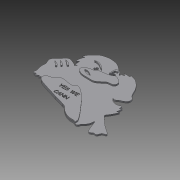
# Autodesk Inventor part: logo
Saved by Autodesk Inventor 2014 SP1 (Build 180222100, 222)
## iProperties
Created: 2015-10-19
Part Number: logo
Material: Generic
Document SubType Name: Modeling
Designer: Clayton
Density: 1 g/cm^3
Appearance: Default
Author: Clayton
Autodesk Inventor part; units mm, degrees
(part 1 of 2)
ref_plane "YZ Plane" through (0, 0, 0) normal (1, 0, 0) x (0, 1, 0)
ref_plane "XZ Plane" through (0, 0, 0) normal (0, 1, 0) x (-1, 0, 0)
ref_plane "XY Plane" through (0, 0, 0) normal (0, 0, 1) x (1, 0, 0)
sketch "Sketch1" plane through (0, 0, 0) normal (0, 1, 0) x (-1, 0, 0)
  line L0 (205.3182, -105.8082) -> (14.8182, -105.8082) construction
  line L1 (14.8182, -105.8082) -> (14.8182, 35.7439) construction
  line L2 (14.8182, 35.7439) -> (205.3182, 35.7439) construction
  line L3 (205.3182, 35.7439) -> (205.3182, -105.8082) construction
  line L4 (119.6658, -99.1182) -> (125.0217, -103.8066) construction
  line L5 (125.0217, -103.8066) -> (133.3036, -105.4948) construction
  line L6 (133.3036, -105.4948) -> (139.5998, -105.8082) construction
  line L7 (139.5998, -105.8082) -> (142.3045, -105.8082) construction
  line L8 (142.3045, -105.8082) -> (145.8288, -105.2062) construction
  line L9 (145.8288, -105.2062) -> (149.5668, -104.1037) construction
  line L10 (149.5668, -104.1037) -> (153.0365, -103.4823) construction
  line L11 (153.0365, -103.4823) -> (156.2624, -101.346) construction
  line L12 (156.2624, -101.346) -> (158.2697, -99.538) construction
  line L13 (158.2697, -99.538) -> (160.1706, -97.7361) construction
  line L14 (160.1706, -97.7361) -> (161.546, -96.1826) construction
  line L15 (161.546, -96.1826) -> (163.2097, -94.5009) construction
  line L16 (163.2097, -94.5009) -> (165.0974, -92.3655) construction
  line L17 (165.0974, -92.3655) -> (166.0638, -91.0856) construction
  line L18 (166.0638, -91.0856) -> (167.5222, -88.5574) construction
  line L19 (167.5222, -88.5574) -> (168.3582, -86.9182) construction
  line L20 (168.3582, -86.9182) -> (169.2598, -85.5249) construction
  line L21 (169.2598, -85.5249) -> (169.4073, -84.6889) construction
  line L22 (169.4073, -84.6889) -> (168.809, -84.5926) construction
  line L23 (168.809, -84.5926) -> (168.0493, -85.2715) construction
  line L24 (168.0493, -85.2715) -> (167.2824, -85.5249) construction
  line L25 (167.2824, -85.5249) -> (166.0912, -85.7774) construction
  line L26 (166.0912, -85.7774) -> (165.3732, -85.7774) construction
  spline S0 degree 4 poles (119.6658, -99.1182) (125.0217, -103.8066) (133.3036, -105.4948) (139.5998, -105.8082) (142.3045, -105.8082) (145.8288, -105.2062) (149.5668, -104.1037) (153.0365, -103.4823) (156.2624, -101.346) (158.2697, -99.538) (160.1706, -97.7361) (161.546, -96.1826) (163.2097, -94.5009) (165.0974, -92.3655) (166.0638, -91.0856) (167.5222, -88.5574) (168.3582, -86.9182) (169.2598, -85.5249) (169.4073, -84.6889) (168.809, -84.5926) (168.0493, -85.2715) (167.2824, -85.5249) (166.0912, -85.7774) (165.3732, -85.7774) knots 1 1 1 1 1 2 3 4 5 6 7 8 9 10 11 12 13 14 15 16 17 18 19 20 21 21 21 21 21
  line L27 (72.0061, 24.2829) -> (70.6525, 24.5535) construction
  line L28 (70.6525, 24.5535) -> (69.4998, 24.2136) construction
  line L29 (69.4998, 24.2136) -> (68.435, 23.4099) construction
  line L30 (68.435, 23.4099) -> (67.5909, 22.3816) construction
  line L31 (67.5909, 22.3816) -> (67.4318, 21.4798) construction
  line L32 (67.4318, 21.4798) -> (67.1775, 20.7659) construction
  line L33 (67.1775, 20.7659) -> (67.1345, 19.9018) construction
  line L34 (67.1345, 19.9018) -> (66.446, 19.2058) construction
  line L35 (66.446, 19.2058) -> (65.2763, 18.0971) construction
  line L36 (65.2763, 18.0971) -> (64.2775, 17.083) construction
  line L37 (64.2775, 17.083) -> (63.0251, 15.817) construction
  line L38 (63.0251, 15.817) -> (62.3988, 14.8491) construction
  line L39 (62.3988, 14.8491) -> (61.8964, 13.8641) construction
  line L40 (61.8964, 13.8641) -> (61.0497, 12.5555) construction
  line L41 (61.0497, 12.5555) -> (60.8463, 11.5383) construction
  line L42 (60.8463, 11.5383) -> (60.3804, 10.6247) construction
  line L43 (60.3804, 10.6247) -> (59.9183, 9.7186) construction
  line L44 (59.9183, 9.7186) -> (59.6793, 8.5233) construction
  line L45 (59.6793, 8.5233) -> (59.6041, 7.0137) construction
  line L46 (59.6041, 7.0137) -> (59.6041, 5.8018) construction
  line L47 (59.6041, 5.8018) -> (59.4165, 4.7385) construction
  line L48 (59.4165, 4.7385) -> (59.1255, 3.9217) construction
  line L49 (59.1255, 3.9217) -> (58.8425, 3.3668) construction
  line L50 (58.8425, 3.3668) -> (58.0971, 3.9787) construction
  line L51 (58.0971, 3.9787) -> (57.5959, 5.0609) construction
  line L52 (57.5959, 5.0609) -> (56.7878, 6.8058) construction
  line L53 (56.7878, 6.8058) -> (56.5067, 8.3755) construction
  line L54 (56.5067, 8.3755) -> (55.8124, 9.8748) construction
  spline S1 degree 4 poles (72.0061, 24.2829) (70.6525, 24.5535) (69.4998, 24.2136) (68.435, 23.4099) (67.5909, 22.3816) (67.4318, 21.4798) (67.1775, 20.7659) (67.1345, 19.9018) (66.446, 19.2058) (65.2763, 18.0971) (64.2775, 17.083) (63.0251, 15.817) (62.3988, 14.8491) (61.8964, 13.8641) (61.0497, 12.5555) (60.8463, 11.5383) (60.3804, 10.6247) (59.9183, 9.7186) (59.6793, 8.5233) (59.6041, 7.0137) (59.6041, 5.8018) (59.4165, 4.7385) (59.1255, 3.9217) (58.8425, 3.3668) (58.0971, 3.9787) (57.5959, 5.0609) (56.7878, 6.8058) (56.5067, 8.3755) (55.8124, 9.8748) knots 1 1 1 1 1 2 3 4 5 6 7 8 9 10 11 12 13 14 15 16 17 18 19 20 21 22 23 24 25 26 26 26 26 26
  line L55 (55.8124, 9.8748) -> (54.8371, 11.9808) construction
  line L56 (54.8371, 11.9808) -> (53.6125, 15.232) construction
  line L57 (53.6125, 15.232) -> (51.641, 19.9262) construction
  line L58 (51.641, 19.9262) -> (50.2656, 22.8961) construction
  line L59 (50.2656, 22.8961) -> (49.1599, 23.99) construction
  line L60 (49.1599, 23.99) -> (47.6368, 24.7667) construction
  line L61 (47.6368, 24.7667) -> (46.3346, 24.5335) construction
  line L62 (46.3346, 24.5335) -> (45.2431, 24.028) construction
  line L63 (45.2431, 24.028) -> (43.9979, 22.5111) construction
  line L64 (43.9979, 22.5111) -> (42.8586, 21.6512) construction
  line L65 (42.8586, 21.6512) -> (41.6778, 21.71) construction
  line L66 (41.6778, 21.71) -> (40.6321, 21.8548) construction
  line L67 (40.6321, 21.8548) -> (39.3449, 22.0819) construction
  line L68 (39.3449, 22.0819) -> (37.9514, 22.1513) construction
  line L69 (37.9514, 22.1513) -> (37.0993, 21.7566) construction
  line L70 (37.0993, 21.7566) -> (36.1467, 20.5961) construction
  line L71 (36.1467, 20.5961) -> (35.8442, 18.8823) construction
  line L72 (35.8442, 18.8823) -> (35.6072, 17.5392) construction
  line L73 (35.6072, 17.5392) -> (34.5467, 15.9002) construction
  line L74 (34.5467, 15.9002) -> (33.8767, 15.084) construction
  line L75 (33.8767, 15.084) -> (32.4017, 14.4009) construction
  line L76 (32.4017, 14.4009) -> (31.3382, 13.9084) construction
  line L77 (31.3382, 13.9084) -> (30.0361, 13.6752) construction
  line L78 (30.0361, 13.6752) -> (29.6443, 13.4938) construction
  line L79 (29.6443, 13.4938) -> (28.91, 12.5992) construction
  line L80 (28.91, 12.5992) -> (28.4728, 11.7419) construction
  line L81 (28.4728, 11.7419) -> (28.751, 11.1411) construction
  line L82 (28.751, 11.1411) -> (29.3294, 10.569) construction
  line L83 (29.3294, 10.569) -> (30.2816, 9.7873) construction
  line L84 (30.2816, 9.7873) -> (31.1945, 9.1966) construction
  spline S2 degree 4 poles (55.8124, 9.8748) (54.8371, 11.9808) (53.6125, 15.232) (51.641, 19.9262) (50.2656, 22.8961) (49.1599, 23.99) (47.6368, 24.7667) (46.3346, 24.5335) (45.2431, 24.028) (43.9979, 22.5111) (42.8586, 21.6512) (41.6778, 21.71) (40.6321, 21.8548) (39.3449, 22.0819) (37.9514, 22.1513) (37.0993, 21.7566) (36.1467, 20.5961) (35.8442, 18.8823) (35.6072, 17.5392) (34.5467, 15.9002) (33.8767, 15.084) (32.4017, 14.4009) (31.3382, 13.9084) (30.0361, 13.6752) (29.6443, 13.4938) (28.91, 12.5992) (28.4728, 11.7419) (28.751, 11.1411) (29.3294, 10.569) (30.2816, 9.7873) (31.1945, 9.1966) knots 1 1 1 1 1 2 3 4 5 6 7 8 9 10 11 12 13 14 15 16 17 18 19 20 21 22 23 24 25 26 27 28 28 28 28 28
  line L85 (31.1945, 9.1966) -> (41.8078, 2.3292) construction
  line L86 (41.8078, 2.3292) -> (46.7072, -2.0019) construction
  spline S3 degree 2 poles (31.1945, 9.1966) (41.8078, 2.3292) (46.7072, -2.0019) knots 1 1 1 2 2 2
  line L87 (46.7072, -2.0019) -> (51.207, -5.9799) construction
  line L88 (51.207, -5.9799) -> (53.5134, -8.2615) construction
  line L89 (53.5134, -8.2615) -> (55.9715, -10.8548) construction
  line L90 (55.9715, -10.8548) -> (58.4698, -13.0633) construction
  line L91 (58.4698, -13.0633) -> (60.1673, -14.7426) construction
  line L92 (60.1673, -14.7426) -> (59.1255, -16.3527) construction
  line L93 (59.1255, -16.3527) -> (57.769, -17.8873) construction
  line L94 (57.769, -17.8873) -> (55.4952, -21.8288) construction
  line L95 (55.4952, -21.8288) -> (53.9817, -24.1678) construction
  line L96 (53.9817, -24.1678) -> (52.5072, -27.5205) construction
  line L97 (52.5072, -27.5205) -> (51.6772, -29.4078) construction
  line L98 (51.6772, -29.4078) -> (50.8092, -31.8445) construction
  line L99 (50.8092, -31.8445) -> (50.6239, -32.8941) construction
  line L100 (50.6239, -32.8941) -> (51.5624, -32.4595) construction
  line L101 (51.5624, -32.4595) -> (52.7167, -31.6951) construction
  line L102 (52.7167, -31.6951) -> (54.3148, -30.839) construction
  line L103 (54.3148, -30.839) -> (54.927, -30.839) construction
  line L104 (54.927, -30.839) -> (54.5168, -32.8908) construction
  line L105 (54.5168, -32.8908) -> (53.7795, -34.9605) construction
  line L106 (53.7795, -34.9605) -> (53.9987, -36.9223) construction
  line L107 (53.9987, -36.9223) -> (53.9987, -39.207) construction
  line L108 (53.9987, -39.207) -> (53.9987, -39.8781) construction
  line L109 (53.9987, -39.8781) -> (54.1947, -40.9729) construction
  line L110 (54.1947, -40.9729) -> (54.9689, -39.7764) construction
  line L111 (54.9689, -39.7764) -> (56.2034, -38.1415) construction
  line L112 (56.2034, -38.1415) -> (57.0827, -37.4778) construction
  line L113 (57.0827, -37.4778) -> (56.9666, -39.8108) construction
  line L114 (56.9666, -39.8108) -> (57.2605, -42.4419) construction
  line L115 (57.2605, -42.4419) -> (57.2605, -44.4702) construction
  line L116 (57.2605, -44.4702) -> (60.64, -42.8559) construction
  line L117 (60.64, -42.8559) -> (62.1808, -42.1423) construction
  spline S4 degree 4 poles (46.7072, -2.0019) (51.207, -5.9799) (53.5134, -8.2615) (55.9715, -10.8548) (58.4698, -13.0633) (60.1673, -14.7426) (59.1255, -16.3527) (57.769, -17.8873) (55.4952, -21.8288) (53.9817, -24.1678) (52.5072, -27.5205) (51.6772, -29.4078) (50.8092, -31.8445) (50.6239, -32.8941) (51.5624, -32.4595) (52.7167, -31.6951) (54.3148, -30.839) (54.927, -30.839) (54.5168, -32.8908) (53.7795, -34.9605) (53.9987, -36.9223) (53.9987, -39.207) (53.9987, -39.8781) (54.1947, -40.9729) (54.9689, -39.7764) (56.2034, -38.1415) (57.0827, -37.4778) (56.9666, -39.8108) (57.2605, -42.4419) (57.2605, -44.4702) (60.64, -42.8559) (62.1808, -42.1423) knots 0 0 0 0 0 1 2 3 4 5 6 7 8 9 10 11 12 13 14 15 16 17 18 19 20 21 22 23 24 25 26 27 28 28 28 28 28
  line L118 (119.6658, -99.1182) -> (118.059, -96.9894) construction
  line L119 (118.059, -96.9894) -> (113.9343, -95.5201) construction
  line L120 (113.9343, -95.5201) -> (111.4066, -93.6115) construction
  line L121 (111.4066, -93.6115) -> (109.8893, -91.6013) construction
  line L122 (109.8893, -91.6013) -> (109.115, -89.9293) construction
  spline S5 degree 4 poles (119.6658, -99.1182) (118.059, -96.9894) (113.9343, -95.5201) (111.4066, -93.6115) (109.8893, -91.6013) (109.115, -89.9293) knots 1 1 1 1 1 2 3 3 3 3 3
  line L123 (109.115, -89.9293) -> (108.5171, -89.1372) construction
  line L124 (108.5171, -89.1372) -> (107.1359, -88.4328) construction
  line L125 (107.1359, -88.4328) -> (105.7977, -88.6724) construction
  line L126 (105.7977, -88.6724) -> (106.6397, -89.4168) construction
  line L127 (106.6397, -89.4168) -> (107.5985, -90.1407) construction
  line L128 (107.5985, -90.1407) -> (108.2479, -90.631) construction
  line L129 (108.2479, -90.631) -> (108.0753, -91.1157) construction
  line L130 (108.0753, -91.1157) -> (107.2685, -91.4545) construction
  spline S6 degree 4 poles (109.115, -89.9293) (108.5171, -89.1372) (107.1359, -88.4328) (105.7977, -88.6724) (106.6397, -89.4168) (107.5985, -90.1407) (108.2479, -90.631) (108.0753, -91.1157) (107.2685, -91.4545) knots 1 1 1 1 1 2 3 4 5 6 6 6 6 6
  line L131 (107.2685, -91.4545) -> (105.7476, -91.7269) construction
  line L132 (105.7476, -91.7269) -> (104.5043, -91.9495) construction
  line L133 (104.5043, -91.9495) -> (102.708, -92.1502) construction
  line L134 (102.708, -92.1502) -> (102.0805, -92.4137) construction
  line L135 (102.0805, -92.4137) -> (102.5235, -93.0007) construction
  line L136 (102.5235, -93.0007) -> (103.1602, -93.4814) construction
  line L137 (103.1602, -93.4814) -> (103.7583, -94.2738) construction
  line L138 (103.7583, -94.2738) -> (105.2444, -95.0317) construction
  line L139 (105.2444, -95.0317) -> (105.8009, -95.2299) construction
  line L140 (105.8009, -95.2299) -> (105.6372, -95.6894) construction
  line L141 (105.6372, -95.6894) -> (104.7195, -95.6894) construction
  line L142 (104.7195, -95.6894) -> (103.6929, -95.8733) construction
  line L143 (103.6929, -95.8733) -> (102.1959, -95.7988) construction
  spline S7 degree 4 poles (107.2685, -91.4545) (105.7476, -91.7269) (104.5043, -91.9495) (102.708, -92.1502) (102.0805, -92.4137) (102.5235, -93.0007) (103.1602, -93.4814) (103.7583, -94.2738) (105.2444, -95.0317) (105.8009, -95.2299) (105.6372, -95.6894) (104.7195, -95.6894) (103.6929, -95.8733) (102.1959, -95.7988) knots 1 1 1 1 1 2 3 4 5 6 7 8 9 10 11 11 11 11 11
  line L144 (102.1959, -95.7988) -> (99.1957, -95.7988) construction
  line L145 (99.1957, -95.7988) -> (95.4586, -95.0516) construction
  line L146 (95.4586, -95.0516) -> (95.7146, -96.4807) construction
  line L147 (95.7146, -96.4807) -> (96.2691, -97.2154) construction
  line L148 (96.2691, -97.2154) -> (97.6123, -97.9004) construction
  line L149 (97.6123, -97.9004) -> (97.6123, -98.5529) construction
  line L150 (97.6123, -98.5529) -> (96.4478, -98.5529) construction
  line L151 (96.4478, -98.5529) -> (94.8687, -97.9004) construction
  line L152 (94.8687, -97.9004) -> (93.2661, -97.5177) construction
  line L153 (93.2661, -97.5177) -> (91.6055, -97.2878) construction
  line L154 (91.6055, -97.2878) -> (90.3146, -96.828) construction
  line L155 (90.3146, -96.828) -> (88.9644, -96.347) construction
  spline S8 degree 4 poles (102.1959, -95.7988) (99.1957, -95.7988) (95.4586, -95.0516) (95.7146, -96.4807) (96.2691, -97.2154) (97.6123, -97.9004) (97.6123, -98.5529) (96.4478, -98.5529) (94.8687, -97.9004) (93.2661, -97.5177) (91.6055, -97.2878) (90.3146, -96.828) (88.9644, -96.347) knots 1 1 1 1 1 2 3 4 5 6 7 8 9 10 10 10 10 10
  line L156 (88.9644, -96.347) -> (86.3766, -95.4252) construction
  line L157 (86.3766, -95.4252) -> (84.6652, -94.1329) construction
  line L158 (84.6652, -94.1329) -> (82.9068, -92.8052) construction
  line L159 (82.9068, -92.8052) -> (80.2742, -90.8175) construction
  line L160 (80.2742, -90.8175) -> (77.1184, -88.0277) construction
  spline S9 degree 4 poles (88.9644, -96.347) (86.3766, -95.4252) (84.6652, -94.1329) (82.9068, -92.8052) (80.2742, -90.8175) (77.1184, -88.0277) knots 1 1 1 1 1 2 3 3 3 3 3
  line L161 (77.1184, -88.0277) -> (75.3437, -85.8783) construction
  line L162 (75.3437, -85.8783) -> (73.6356, -83.6153) construction
  line L163 (73.6356, -83.6153) -> (71.9418, -81.0577) construction
  spline S10 degree 3 poles (77.1184, -88.0277) (75.3437, -85.8783) (73.6356, -83.6153) (71.9418, -81.0577) knots 1 1 1 1 2 2 2 2
  line L164 (71.9418, -81.0577) -> (70.0657, -77.5557) construction
  line L165 (70.0657, -77.5557) -> (68.7436, -74.4077) construction
  line L166 (68.7436, -74.4077) -> (67.1241, -70.9107) construction
  line L167 (67.1241, -70.9107) -> (65.1576, -68.3053) construction
  line L168 (65.1576, -68.3053) -> (63.1619, -66.5411) construction
  spline S11 degree 4 poles (71.9418, -81.0577) (70.0657, -77.5557) (68.7436, -74.4077) (67.1241, -70.9107) (65.1576, -68.3053) (63.1619, -66.5411) knots 1 1 1 1 1 2 3 3 3 3 3
  line L169 (63.1619, -66.5411) -> (61.1891, -64.7971) construction
  line L170 (61.1891, -64.7971) -> (59.9079, -63.6645) construction
  line L171 (59.9079, -63.6645) -> (59.3082, -62.3696) construction
  line L172 (59.3082, -62.3696) -> (59.1299, -60.7738) construction
  line L173 (59.1299, -60.7738) -> (59.1299, -59.5702) construction
  line L174 (59.1299, -59.5702) -> (59.2057, -58.0481) construction
  line L175 (59.2057, -58.0481) -> (59.9984, -56.823) construction
  line L176 (59.9984, -56.823) -> (60.3595, -55.8093) construction
  line L177 (60.3595, -55.8093) -> (61.6175, -54.7706) construction
  line L178 (61.6175, -54.7706) -> (62.792, -53.8841) construction
  line L179 (62.792, -53.8841) -> (64.5454, -52.9448) construction
  spline S12 degree 4 poles (63.1619, -66.5411) (61.1891, -64.7971) (59.9079, -63.6645) (59.3082, -62.3696) (59.1299, -60.7738) (59.1299, -59.5702) (59.2057, -58.0481) (59.9984, -56.823) (60.3595, -55.8093) (61.6175, -54.7706) (62.792, -53.8841) (64.5454, -52.9448) knots 1 1 1 1 1 2 3 4 5 6 7 8 9 9 9 9 9
  line L180 (64.5454, -52.9448) -> (65.9669, -52.0034) construction
  line L181 (65.9669, -52.0034) -> (67.5806, -51.5274) construction
  line L182 (67.5806, -51.5274) -> (69.0927, -50.8271) construction
  line L183 (69.0927, -50.8271) -> (70.1695, -50.0144) construction
  line L184 (70.1695, -50.0144) -> (71.2052, -49.2327) construction
  line L185 (71.2052, -49.2327) -> (72.3639, -48.276) construction
  line L186 (72.3639, -48.276) -> (73.336, -47.5423) construction
  line L187 (73.336, -47.5423) -> (74.5879, -47.173) construction
  line L188 (74.5879, -47.173) -> (75.73, -47.2298) construction
  line L189 (75.73, -47.2298) -> (76.7089, -47.5786) construction
  line L190 (76.7089, -47.5786) -> (77.5877, -48.1472) construction
  spline S13 degree 4 poles (64.5454, -52.9448) (65.9669, -52.0034) (67.5806, -51.5274) (69.0927, -50.8271) (70.1695, -50.0144) (71.2052, -49.2327) (72.3639, -48.276) (73.336, -47.5423) (74.5879, -47.173) (75.73, -47.2298) (76.7089, -47.5786) (77.5877, -48.1472) knots 1 1 1 1 1 2 3 4 5 6 7 8 9 9 9 9 9
  line L191 (62.1808, -42.1423) -> (65.9773, -41.0225) construction
  line L192 (65.9773, -41.0225) -> (70.1799, -42.0263) construction
  line L193 (70.1799, -42.0263) -> (73.3464, -43.1542) construction
  line L194 (73.3464, -43.1542) -> (75.6669, -45.2056) construction
  line L195 (75.6669, -45.2056) -> (77.2719, -46.7934) construction
  line L196 (77.2719, -46.7934) -> (78.0678, -47.8479) construction
  line L197 (78.0678, -47.8479) -> (78.0678, -48.1324) construction
  line L198 (78.0678, -48.1324) -> (77.7223, -48.2343) construction
  line L199 (77.7223, -48.2343) -> (77.5877, -48.1472) construction
  spline S14 degree 4 poles (62.1808, -42.1423) (65.9773, -41.0225) (70.1799, -42.0263) (73.3464, -43.1542) (75.6669, -45.2056) (77.2719, -46.7934) (78.0678, -47.8479) (78.0678, -48.1324) (77.7223, -48.2343) (77.5877, -48.1472) knots 1 1 1 1 1 2 3 4 5 6 7 7 7 7 7
  line L200 (72.0061, 24.2829) -> (73.3464, 23.4157) construction
  line L201 (73.3464, 23.4157) -> (75.6669, 22.589) construction
  line L202 (75.6669, 22.589) -> (76.4694, 22.0698) construction
  line L203 (76.4694, 22.0698) -> (78.0678, 22.0698) construction
  line L204 (78.0678, 22.0698) -> (81.9397, 22.0698) construction
  line L205 (81.9397, 22.0698) -> (84.2511, 22.0698) construction
  line L206 (84.2511, 22.0698) -> (87.6705, 21.2531) construction
  line L207 (87.6705, 21.2531) -> (90.3146, 20.3112) construction
  line L208 (90.3146, 20.3112) -> (94.8687, 18.4294) construction
  line L209 (94.8687, 18.4294) -> (97.6123, 16.6542) construction
  line L210 (97.6123, 16.6542) -> (101.7979, 13.4938) construction
  line L211 (101.7979, 13.4938) -> (104.7195, 10.6035) construction
  line L212 (104.7195, 10.6035) -> (107.2685, 8.3502) construction
  line L213 (107.2685, 8.3502) -> (108.0753, 7.8281) construction
  line L214 (108.0753, 7.8281) -> (109.8893, 7.1819) construction
  line L215 (109.8893, 7.1819) -> (112.6705, 6.5177) construction
  spline S15 degree 4 poles (72.0061, 24.2829) (73.3464, 23.4157) (75.6669, 22.589) (76.4694, 22.0698) (78.0678, 22.0698) (81.9397, 22.0698) (84.2511, 22.0698) (87.6705, 21.2531) (90.3146, 20.3112) (94.8687, 18.4294) (97.6123, 16.6542) (101.7979, 13.4938) (104.7195, 10.6035) (107.2685, 8.3502) (108.0753, 7.8281) (109.8893, 7.1819) (112.6705, 6.5177) knots 1 1 1 1 1 2 3 4 5 6 7 8 9 10 11 12 13 14 14 14 14 14
  line L216 (112.6705, 6.5177) -> (116.4732, 5.1631) construction
  line L217 (116.4732, 5.1631) -> (122.8568, 3.6384) construction
  line L218 (122.8568, 3.6384) -> (128.5229, 2.0136) construction
  spline S16 degree 3 poles (112.6705, 6.5177) (116.4732, 5.1631) (122.8568, 3.6384) (128.5229, 2.0136) knots 1 1 1 1 2 2 2 2
  line L219 (128.5229, 2.0136) -> (133.408, 0.448) construction
  line L220 (133.408, 0.448) -> (137.5642, -1.0325) construction
  line L221 (137.5642, -1.0325) -> (144.0666, -2.897) construction
  line L222 (144.0666, -2.897) -> (150.8595, -4.8448) construction
  line L223 (150.8595, -4.8448) -> (156.3592, -6.8039) construction
  line L224 (156.3592, -6.8039) -> (161.9348, -8.4027) construction
  line L225 (161.9348, -8.4027) -> (166.1802, -10.5679) construction
  spline S17 degree 4 poles (128.5229, 2.0136) (133.408, 0.448) (137.5642, -1.0325) (144.0666, -2.897) (150.8595, -4.8448) (156.3592, -6.8039) (161.9348, -8.4027) (166.1802, -10.5679) knots 1 1 1 1 1 2 3 4 5 5 5 5 5
  line L226 (166.1802, -10.5679) -> (169.1501, -12.4896) construction
  line L227 (169.1501, -12.4896) -> (170.815, -14.1366) construction
  line L228 (170.815, -14.1366) -> (171.1441, -17.0833) construction
  line L229 (171.1441, -17.0833) -> (170.5284, -19.2307) construction
  line L230 (170.5284, -19.2307) -> (169.4313, -21.3818) construction
  line L231 (169.4313, -21.3818) -> (167.6803, -21.8983) construction
  line L232 (167.6803, -21.8983) -> (165.3841, -22.9617) construction
  line L233 (165.3841, -22.9617) -> (162.6103, -23.2715) construction
  line L234 (162.6103, -23.2715) -> (160.0581, -24.0243) construction
  line L235 (160.0581, -24.0243) -> (159.147, -24.0243) construction
  spline S18 degree 4 poles (166.1802, -10.5679) (169.1501, -12.4896) (170.815, -14.1366) (171.1441, -17.0833) (170.5284, -19.2307) (169.4313, -21.3818) (167.6803, -21.8983) (165.3841, -22.9617) (162.6103, -23.2715) (160.0581, -24.0243) (159.147, -24.0243) knots 1 1 1 1 1 2 3 4 5 6 7 8 8 8 8 8
  line L236 (159.147, -24.0243) -> (158.507, -24.6712) construction
  line L237 (158.507, -24.6712) -> (157.9485, -25.2358) construction
  line L238 (157.9485, -25.2358) -> (158.3016, -26.4328) construction
  line L239 (158.3016, -26.4328) -> (158.9723, -27.3215) construction
  line L240 (158.9723, -27.3215) -> (159.7617, -27.3215) construction
  line L241 (159.7617, -27.3215) -> (160.5355, -26.7374) construction
  line L242 (160.5355, -26.7374) -> (161.9667, -26.3152) construction
  line L243 (161.9667, -26.3152) -> (163.9423, -25.4855) construction
  line L244 (163.9423, -25.4855) -> (164.994, -25.4855) construction
  line L245 (164.994, -25.4855) -> (166.5641, -25.3101) construction
  line L246 (166.5641, -25.3101) -> (168.5064, -25.3101) construction
  line L247 (168.5064, -25.3101) -> (169.4633, -24.867) construction
  line L248 (169.4633, -24.867) -> (169.7328, -23.9269) construction
  line L249 (169.7328, -23.9269) -> (170.3522, -22.9696) construction
  line L250 (170.3522, -22.9696) -> (170.7667, -22.157) construction
  line L251 (170.7667, -22.157) -> (171.6798, -20.7458) construction
  spline S19 degree 4 poles (159.147, -24.0243) (158.507, -24.6712) (157.9485, -25.2358) (158.3016, -26.4328) (158.9723, -27.3215) (159.7617, -27.3215) (160.5355, -26.7374) (161.9667, -26.3152) (163.9423, -25.4855) (164.994, -25.4855) (166.5641, -25.3101) (168.5064, -25.3101) (169.4633, -24.867) (169.7328, -23.9269) (170.3522, -22.9696) (170.7667, -22.157) (171.6798, -20.7458) knots 1 1 1 1 1 2 3 4 5 6 7 8 9 10 11 12 13 14 14 14 14 14
  line L252 (171.6798, -20.7458) -> (172.6602, -19.2307) construction
  line L253 (172.6602, -19.2307) -> (173.7224, -18.157) construction
  line L254 (173.7224, -18.157) -> (175.1449, -17.0833) construction
  line L255 (175.1449, -17.0833) -> (176.5792, -16.0007) construction
  line L256 (176.5792, -16.0007) -> (177.311, -15.6618) construction
  line L257 (177.311, -15.6618) -> (177.311, -16.5124) construction
  line L258 (177.311, -16.5124) -> (177.311, -18.047) construction
  spline S20 degree 4 poles (171.6798, -20.7458) (172.6602, -19.2307) (173.7224, -18.157) (175.1449, -17.0833) (176.5792, -16.0007) (177.311, -15.6618) (177.311, -16.5124) (177.311, -18.047) knots 1 1 1 1 1 2 3 4 5 5 5 5 5
  line L259 (177.311, -18.047) -> (177.5443, -18.5507) construction
  line L260 (177.5443, -18.5507) -> (178.2116, -18.047) construction
  line L261 (178.2116, -18.047) -> (179.3702, -17.2797) construction
  line L262 (179.3702, -17.2797) -> (180.9269, -16.5588) construction
  line L263 (180.9269, -16.5588) -> (182.49, -16.0977) construction
  line L264 (182.49, -16.0977) -> (183.639, -15.7588) construction
  line L265 (183.639, -15.7588) -> (184.3149, -15.7588) construction
  line L266 (184.3149, -15.7588) -> (184.4099, -16.6095) construction
  line L267 (184.4099, -16.6095) -> (183.8452, -17.1803) construction
  line L268 (183.8452, -17.1803) -> (183.2216, -18.144) construction
  line L269 (183.2216, -18.144) -> (183.2216, -18.7909) construction
  line L270 (183.2216, -18.7909) -> (184.1723, -19.0635) construction
  line L271 (184.1723, -19.0635) -> (184.7275, -18.5023) construction
  line L272 (184.7275, -18.5023) -> (185.7032, -18.2145) construction
  line L273 (185.7032, -18.2145) -> (187.1504, -17.7876) construction
  line L274 (187.1504, -17.7876) -> (188.1246, -18.0203) construction
  line L275 (188.1246, -18.0203) -> (189.1318, -18.0203) construction
  line L276 (189.1318, -18.0203) -> (188.9205, -18.7573) construction
  line L277 (188.9205, -18.7573) -> (188.6354, -19.7516) construction
  line L278 (188.6354, -19.7516) -> (188.2586, -20.8093) construction
  line L279 (188.2586, -20.8093) -> (187.9215, -22.2204) construction
  line L280 (187.9215, -22.2204) -> (188.0881, -23.7114) construction
  line L281 (188.0881, -23.7114) -> (188.0881, -25.017) construction
  line L282 (188.0881, -25.017) -> (188.6402, -26.2091) construction
  line L283 (188.6402, -26.2091) -> (189.3205, -30.008) construction
  line L284 (189.3205, -30.008) -> (190.4389, -33.8) construction
  line L285 (190.4389, -33.8) -> (190.4389, -36.1743) construction
  line L286 (190.4389, -36.1743) -> (190.0104, -39.2705) construction
  line L287 (190.0104, -39.2705) -> (190.0104, -41.5879) construction
  line L288 (190.0104, -41.5879) -> (190.3933, -43.7265) construction
  line L289 (190.3933, -43.7265) -> (191.7395, -45.7591) construction
  line L290 (191.7395, -45.7591) -> (192.4883, -48.2978) construction
  line L291 (192.4883, -48.2978) -> (193.4038, -50.2747) construction
  spline S21 degree 4 poles (177.311, -18.047) (177.5443, -18.5507) (178.2116, -18.047) (179.3702, -17.2797) (180.9269, -16.5588) (182.49, -16.0977) (183.639, -15.7588) (184.3149, -15.7588) (184.4099, -16.6095) (183.8452, -17.1803) (183.2216, -18.144) (183.2216, -18.7909) (184.1723, -19.0635) (184.7275, -18.5023) (185.7032, -18.2145) (187.1504, -17.7876) (188.1246, -18.0203) (189.1318, -18.0203) (188.9205, -18.7573) (188.6354, -19.7516) (188.2586, -20.8093) (187.9215, -22.2204) (188.0881, -23.7114) (188.0881, -25.017) (188.6402, -26.2091) (189.3205, -30.008) (190.4389, -33.8) (190.4389, -36.1743) (190.0104, -39.2705) (190.0104, -41.5879) (190.3933, -43.7265) (191.7395, -45.7591) (192.4883, -48.2978) (193.4038, -50.2747) knots 1 1 1 1 1 2 3 4 5 6 7 8 9 10 11 12 13 14 15 16 17 18 19 20 21 22 23 24 25 26 27 28 29 30 31 31 31 31 31
  line L292 (193.4038, -50.2747) -> (193.4038, -53.8841) construction
  line L293 (193.4038, -53.8841) -> (190.4389, -56.8811) construction
  line L294 (190.4389, -56.8811) -> (188.7998, -59.4143) construction
  line L295 (188.7998, -59.4143) -> (185.0348, -61.9077) construction
  line L296 (185.0348, -61.9077) -> (182.3095, -66.1196) construction
  line L297 (182.3095, -66.1196) -> (179.5393, -68.9198) construction
  line L298 (179.5393, -68.9198) -> (176.7249, -70.2232) construction
  spline S22 degree 4 poles (193.4038, -50.2747) (193.4038, -53.8841) (190.4389, -56.8811) (188.7998, -59.4143) (185.0348, -61.9077) (182.3095, -66.1196) (179.5393, -68.9198) (176.7249, -70.2232) knots 1 1 1 1 1 2 3 4 5 5 5 5 5
  line L299 (176.7249, -70.2232) -> (175.6404, -70.289) construction
  line L300 (175.6404, -70.289) -> (173.1913, -69.5041) construction
  line L301 (173.1913, -69.5041) -> (169.7328, -68.3957) construction
  line L302 (169.7328, -68.3957) -> (166.9613, -67.2505) construction
  line L303 (166.9613, -67.2505) -> (164.994, -66.4376) construction
  line L304 (164.994, -66.4376) -> (163.5889, -65.3767) construction
  line L305 (163.5889, -65.3767) -> (162.4306, -64.2308) construction
  spline S23 degree 4 poles (176.7249, -70.2232) (175.6404, -70.289) (173.1913, -69.5041) (169.7328, -68.3957) (166.9613, -67.2505) (164.994, -66.4376) (163.5889, -65.3767) (162.4306, -64.2308) knots 1 1 1 1 1 2 3 4 5 5 5 5 5
  line L306 (165.3732, -85.7774) -> (164.8487, -85.7774) construction
  line L307 (164.8487, -85.7774) -> (165.198, -84.932) construction
  line L308 (165.198, -84.932) -> (166.1802, -83.0061) construction
  line L309 (166.1802, -83.0061) -> (166.9613, -81.1158) construction
  spline S24 degree 4 poles (165.3732, -85.7774) (164.8487, -85.7774) (165.198, -84.932) (166.1802, -83.0061) (166.9613, -81.1158) knots 1 1 1 1 1 2 2 2 2 2
  line L310 (166.9613, -81.1158) -> (167.6803, -78.8725) construction
  line L311 (167.6803, -78.8725) -> (167.6803, -74.9282) construction
  line L312 (167.6803, -74.9282) -> (167.5222, -72.325) construction
  line L313 (167.5222, -72.325) -> (167.2444, -72.0502) construction
  line L314 (167.2444, -72.0502) -> (166.7335, -72.5667) construction
  line L315 (166.7335, -72.5667) -> (166.1802, -73.2994) construction
  line L316 (166.1802, -73.2994) -> (165.2381, -74.2517) construction
  line L317 (165.2381, -74.2517) -> (164.4681, -74.6642) construction
  line L318 (164.4681, -74.6642) -> (163.7003, -74.9534) construction
  line L319 (163.7003, -74.9534) -> (163.4827, -74.6248) construction
  line L320 (163.4827, -74.6248) -> (163.4276, -73.717) construction
  line L321 (163.4276, -73.717) -> (163.4276, -69.8966) construction
  line L322 (163.4276, -69.8966) -> (162.881, -66.8441) construction
  spline S25 degree 4 poles (166.9613, -81.1158) (167.6803, -78.8725) (167.6803, -74.9282) (167.5222, -72.325) (167.2444, -72.0502) (166.7335, -72.5667) (166.1802, -73.2994) (165.2381, -74.2517) (164.4681, -74.6642) (163.7003, -74.9534) (163.4827, -74.6248) (163.4276, -73.717) (163.4276, -69.8966) (162.881, -66.8441) knots 1 1 1 1 1 2 3 4 5 6 7 8 9 10 11 11 11 11 11
  line L323 (162.881, -66.8441) -> (162.4384, -65.6691) construction
  line L324 (162.4384, -65.6691) -> (161.6049, -66.2211) construction
  line L325 (161.6049, -66.2211) -> (160.2253, -67.1348) construction
  spline S26 degree 3 poles (162.881, -66.8441) (162.4384, -65.6691) (161.6049, -66.2211) (160.2253, -67.1348) knots 1 1 1 1 2 2 2 2
  line L326 (160.2253, -67.1348) -> (159.147, -67.1348) construction
  line L327 (159.147, -67.1348) -> (159.8367, -66.4376) construction
  line L328 (159.8367, -66.4376) -> (160.6377, -65.3767) construction
  line L329 (160.6377, -65.3767) -> (161.7713, -64.2308) construction
  line L330 (161.7713, -64.2308) -> (162.4306, -64.2308) construction
  spline S27 degree 4 poles (160.2253, -67.1348) (159.147, -67.1348) (159.8367, -66.4376) (160.6377, -65.3767) (161.7713, -64.2308) (162.4306, -64.2308) knots 1 1 1 1 1 2 3 3 3 3 3
  point P0 (0, 0)
  constraints: 153 parallel, 101 perpendicular, 6 collinear, 4 point on line, 86 other
extrude "Extrusion1" add sketch "Sketch1" along normal blind 2.54
sketch "Sketch2" plane through (0, 2.54, 0) normal (0, 1, 0) x (1, 0, 0)
  line L0 (-205.4862, 105.9068) -> (-14.9862, 105.9068) construction
  line L1 (-14.9862, 105.9068) -> (-14.9862, -35.6452) construction
  line L2 (-14.9862, -35.6452) -> (-205.4862, -35.6452) construction
  line L3 (-205.4862, -35.6452) -> (-205.4862, 105.9068) construction
  line L4 (-139.7824, 80.7529) -> (-139.2931, 80.2473) construction
  line L5 (-139.2931, 80.2473) -> (-138.706, 79.4481) construction
  line L6 (-138.706, 79.4481) -> (-138.1188, 78.8121) construction
  line L7 (-138.1188, 78.8121) -> (-138.5592, 78.6163) construction
  line L8 (-138.5592, 78.6163) -> (-139.6356, 78.8447) construction
  line L9 (-139.6356, 78.8447) -> (-140.5326, 78.9752) construction
  line L10 (-140.5326, 78.9752) -> (-140.9567, 78.6653) construction
  line L11 (-140.9567, 78.6653) -> (-140.8751, 77.9313) construction
  line L12 (-140.8751, 77.9313) -> (-140.8751, 76.9202) construction
  line L13 (-140.8751, 76.9202) -> (-140.1901, 76.0231) construction
  line L14 (-140.1901, 76.0231) -> (-139.5704, 75.4849) construction
  line L15 (-139.5704, 75.4849) -> (-138.3472, 74.7836) construction
  line L16 (-138.3472, 74.7836) -> (-137.0098, 74.9793) construction
  line L17 (-137.0098, 74.9793) -> (-136.2595, 75.7296) construction
  line L18 (-136.2595, 75.7296) -> (-135.4278, 76.2352) construction
  line L19 (-135.4278, 76.2352) -> (-134.7591, 76.9854) construction
  line L20 (-134.7591, 76.9854) -> (-134.5797, 77.8987) construction
  line L21 (-134.5797, 77.8987) -> (-134.7265, 79.1872) construction
  line L22 (-134.7265, 79.1872) -> (-135.1505, 79.9374) construction
  line L23 (-135.1505, 79.9374) -> (-135.4767, 80.5898) construction
  line L24 (-135.4767, 80.5898) -> (-136.3574, 81.1158) construction
  line L25 (-136.3574, 81.1158) -> (-136.9445, 81.4705) construction
  line L26 (-136.9445, 81.4705) -> (-138.0699, 81.4705) construction
  line L27 (-138.0699, 81.4705) -> (-138.8038, 81.0577) construction
  line L28 (-138.8038, 81.0577) -> (-139.7824, 80.7529) construction
  spline S0 degree 4 poles (-139.7824, 80.7529) (-139.2931, 80.2473) (-138.706, 79.4481) (-138.1188, 78.8121) (-138.5592, 78.6163) (-139.6356, 78.8447) (-140.5326, 78.9752) (-140.9567, 78.6653) (-140.8751, 77.9313) (-140.8751, 76.9202) (-140.1901, 76.0231) (-139.5704, 75.4849) (-138.3472, 74.7836) (-137.0098, 74.9793) (-136.2595, 75.7296) (-135.4278, 76.2352) (-134.7591, 76.9854) (-134.5797, 77.8987) (-134.7265, 79.1872) (-135.1505, 79.9374) (-135.4767, 80.5898) (-136.3574, 81.1158) (-136.9445, 81.4705) (-138.0699, 81.4705) (-138.8038, 81.0577) (-139.7824, 80.7529) knots 1 1 1 1 1 2 3 4 5 6 7 8 9 10 11 12 13 14 15 16 17 18 19 20 21 22 23 23 23 23 23
  line L29 (-112.1882, 86.8255) -> (-112.1882, 85.9945) construction
  line L30 (-112.1882, 85.9945) -> (-112.2998, 85.4264) construction
  line L31 (-112.2998, 85.4264) -> (-112.2998, 84.7601) construction
  line L32 (-112.2998, 84.7601) -> (-112.1805, 84.3771) construction
  line L33 (-112.1805, 84.3771) -> (-111.4587, 84.9283) construction
  line L34 (-111.4587, 84.9283) -> (-110.6689, 85.3726) construction
  line L35 (-110.6689, 85.3726) -> (-110.2362, 85.1112) construction
  line L36 (-110.2362, 85.1112) -> (-110.0361, 84.4685) construction
  line L37 (-110.0361, 84.4685) -> (-110.1694, 83.7895) construction
  line L38 (-110.1694, 83.7895) -> (-110.0579, 82.8108) construction
  line L39 (-110.0579, 82.8108) -> (-110.2362, 82.133) construction
  line L40 (-110.2362, 82.133) -> (-110.679, 81.4003) construction
  line L41 (-110.679, 81.4003) -> (-111.559, 80.9053) construction
  line L42 (-111.559, 80.9053) -> (-112.4931, 80.678) construction
  line L43 (-112.4931, 80.678) -> (-113.2672, 80.5898) construction
  line L44 (-113.2672, 80.5898) -> (-114.0975, 80.7529) construction
  line L45 (-114.0975, 80.7529) -> (-115.0415, 81.5943) construction
  line L46 (-115.0415, 81.5943) -> (-115.6666, 82.4129) construction
  line L47 (-115.6666, 82.4129) -> (-115.5434, 84.9785) construction
  line L48 (-115.5434, 84.9785) -> (-115.4089, 85.6629) construction
  line L49 (-115.4089, 85.6629) -> (-114.374, 86.6978) construction
  line L50 (-114.374, 86.6978) -> (-113.8381, 86.8647) construction
  line L51 (-113.8381, 86.8647) -> (-112.9202, 86.9693) construction
  line L52 (-112.9202, 86.9693) -> (-112.1882, 86.8255) construction
  spline S1 degree 4 poles (-112.1882, 86.8255) (-112.1882, 85.9945) (-112.2998, 85.4264) (-112.2998, 84.7601) (-112.1805, 84.3771) (-111.4587, 84.9283) (-110.6689, 85.3726) (-110.2362, 85.1112) (-110.0361, 84.4685) (-110.1694, 83.7895) (-110.0579, 82.8108) (-110.2362, 82.133) (-110.679, 81.4003) (-111.559, 80.9053) (-112.4931, 80.678) (-113.2672, 80.5898) (-114.0975, 80.7529) (-115.0415, 81.5943) (-115.6666, 82.4129) (-115.5434, 84.9785) (-115.4089, 85.6629) (-114.374, 86.6978) (-113.8381, 86.8647) (-112.9202, 86.9693) (-112.1882, 86.8255) knots 1 1 1 1 1 2 3 4 5 6 7 8 9 10 11 12 13 14 15 16 17 18 19 20 21 22 22 22 22 22
  point P0 (0, 0)
  constraints: 14 parallel, 9 perpendicular, 7 other
extrude "Extrusion2" cut sketch "Sketch2" against normal blind 2.54
sketch "Sketch3" plane through (0, 2.54, 0) normal (0, 1, 0) x (1, 0, 0)
  line L0 (-205.4341, 105.7807) -> (-14.9341, 105.7807) construction
  line L1 (-14.9341, 105.7807) -> (-14.9341, -35.7714) construction
  line L2 (-14.9341, -35.7714) -> (-205.4341, -35.7714) construction
  line L3 (-205.4341, -35.7714) -> (-205.4341, 105.7807) construction
  line L4 (-100.2607, 79.2979) -> (-107.2685, 82.9136) construction
  line L5 (-107.2685, 82.9136) -> (-108.7646, 80.3498) construction
  line L6 (-108.7646, 80.3498) -> (-112.1882, 78.2461) construction
  line L7 (-112.1882, 78.2461) -> (-118.1655, 76.7341) construction
  line L8 (-118.1655, 76.7341) -> (-123.4247, 76.0767) construction
  line L9 (-123.4247, 76.0767) -> (-129.6042, 75.485) construction
  line L10 (-129.6042, 75.485) -> (-132.4968, 74.6304) construction
  line L11 (-132.4968, 74.6304) -> (-133.6801, 73.5786) construction
  line L12 (-133.6801, 73.5786) -> (-133.6801, 71.8693) construction
  line L13 (-133.6801, 71.8693) -> (-135.6523, 71.2119) construction
  line L14 (-135.6523, 71.2119) -> (-137.6245, 71.2119) construction
  line L15 (-137.6245, 71.2119) -> (-141.7661, 70.2232) construction
  line L16 (-141.7661, 70.2232) -> (-145.4475, 69.3055) construction
  line L17 (-145.4475, 69.3055) -> (-148.3401, 66.5411) construction
  line L18 (-148.3401, 66.5411) -> (-150.3123, 64.2308) construction
  line L19 (-150.3123, 64.2308) -> (-150.3123, 60.9565) construction
  line L20 (-150.3123, 60.9565) -> (-147.4197, 58.1297) construction
  line L21 (-147.4197, 58.1297) -> (-142.4892, 55.8288) construction
  line L22 (-142.4892, 55.8288) -> (-138.1784, 55.0936) construction
  line L23 (-138.1784, 55.0936) -> (-136.6438, 55.0485) construction
  line L24 (-136.6438, 55.0485) -> (-134.5141, 54.7383) construction
  line L25 (-134.5141, 54.7383) -> (-133.5825, 54.9321) construction
  line L26 (-133.5825, 54.9321) -> (-132.6857, 54.9321) construction
  line L27 (-132.6857, 54.9321) -> (-129.4722, 54.9321) construction
  line L28 (-129.4722, 54.9321) -> (-124.4809, 54.5417) construction
  line L29 (-124.4809, 54.5417) -> (-122.9461, 54.8353) construction
  line L30 (-122.9461, 54.8353) -> (-121.479, 54.6692) construction
  line L31 (-121.479, 54.6692) -> (-118.3787, 55.1951) construction
  line L32 (-118.3787, 55.1951) -> (-115.7489, 56.8283) construction
  line L33 (-115.7489, 56.8283) -> (-112.1882, 59.4857) construction
  line L34 (-112.1882, 59.4857) -> (-109.4375, 62.1432) construction
  line L35 (-109.4375, 62.1432) -> (-106.1711, 64.9113) construction
  line L36 (-106.1711, 64.9113) -> (-104.0525, 65.7262) construction
  line L37 (-104.0525, 65.7262) -> (-101.8316, 65.7216) construction
  line L38 (-101.8316, 65.7216) -> (-100.9919, 65.8275) construction
  line L39 (-100.9919, 65.8275) -> (-100.9919, 65.7262) construction
  line L40 (-100.9919, 65.7262) -> (-100.2607, 66.0368) construction
  line L41 (-100.2607, 66.0368) -> (-99.1289, 66.0368) construction
  line L42 (-99.1289, 66.0368) -> (-97.6245, 66.0368) construction
  line L43 (-97.6245, 66.0368) -> (-96.9998, 66.5411) construction
  line L44 (-96.9998, 66.5411) -> (-95.8022, 67.1348) construction
  line L45 (-95.8022, 67.1348) -> (-94.6381, 67.9233) construction
  line L46 (-94.6381, 67.9233) -> (-93.8603, 69.3055) construction
  line L47 (-93.8603, 69.3055) -> (-93.8603, 71.8837) construction
  line L48 (-93.8603, 71.8837) -> (-93.8603, 73.494) construction
  line L49 (-93.8603, 73.494) -> (-94.6381, 75.485) construction
  spline S0 degree 4 poles (-100.2607, 79.2979) (-107.2685, 82.9136) (-108.7646, 80.3498) (-112.1882, 78.2461) (-118.1655, 76.7341) (-123.4247, 76.0767) (-129.6042, 75.485) (-132.4968, 74.6304) (-133.6801, 73.5786) (-133.6801, 71.8693) (-135.6523, 71.2119) (-137.6245, 71.2119) (-141.7661, 70.2232) (-145.4475, 69.3055) (-148.3401, 66.5411) (-150.3123, 64.2308) (-150.3123, 60.9565) (-147.4197, 58.1297) (-142.4892, 55.8288) (-138.1784, 55.0936) (-136.6438, 55.0485) (-134.5141, 54.7383) (-133.5825, 54.9321) (-132.6857, 54.9321) (-129.4722, 54.9321) (-124.4809, 54.5417) (-122.9461, 54.8353) (-121.479, 54.6692) (-118.3787, 55.1951) (-115.7489, 56.8283) (-112.1882, 59.4857) (-109.4375, 62.1432) (-106.1711, 64.9113) (-104.0525, 65.7262) (-101.8316, 65.7216) (-100.9919, 65.8275) (-100.9919, 65.7262) (-100.2607, 66.0368) (-99.1289, 66.0368) (-97.6245, 66.0368) (-96.9998, 66.5411) (-95.8022, 67.1348) (-94.6381, 67.9233) (-93.8603, 69.3055) (-93.8603, 71.8837) (-93.8603, 73.494) (-94.6381, 75.485) (-96.9998, 77.6333) (-100.2575, 79.2963) (-100.2607, 79.2979) knots 1 1 1 1 1 2 3 4 5 6 7 8 9 10 11 12 13 14 15 16 17 18 19 20 21 22 23 24 25 26 27 28 29 30 31 32 33 34 35 36 37 38 39 40 41 42 43 44 45 46 46.537582 46.537582 46.537582 46.537582 46.537582
  line L50 (-94.6381, 75.485) -> (-96.9998, 77.6333) construction
  line L51 (-96.9998, 77.6333) -> (-100.2607, 79.2979) construction
  point P0 (-112.1882, 86.8255)
  point P1 (-139.7824, 80.7529)
  point P2 (0, 0)
  constraints: 6 parallel, 2 coincident, 1 point on line, 4 other
extrude "Extrusion3" add sketch "Sketch3" along normal blind 2.54
sketch "Sketch4" plane through (0, 5.08, 0) normal (0, 1, 0) x (1, 0, 0)
  line L0 (-205.2384, 105.7501) -> (-14.7385, 105.7501) construction
  line L1 (-14.7385, 105.7501) -> (-14.7385, -35.802) construction
  line L2 (-14.7385, -35.802) -> (-205.2384, -35.802) construction
  line L3 (-205.2384, -35.802) -> (-205.2384, 105.7501) construction
  line L4 (-130.3466, 60.4688) -> (-131.8592, 61.67) construction
  line L5 (-131.8592, 61.67) -> (-134.662, 63.4496) construction
  line L6 (-134.662, 63.4496) -> (-137.4648, 64.7842) construction
  line L7 (-137.4648, 64.7842) -> (-139.2888, 65.4071) construction
  line L8 (-139.2888, 65.4071) -> (-141.5577, 65.6295) construction
  line L9 (-141.5577, 65.6295) -> (-144.2716, 65.2736) construction
  line L10 (-144.2716, 65.2736) -> (-144.6275, 64.4728) construction
  line L11 (-144.6275, 64.4728) -> (-142.581, 62.7378) construction
  line L12 (-142.581, 62.7378) -> (-139.3333, 61.0472) construction
  line L13 (-139.3333, 61.0472) -> (-136.0856, 59.9795) construction
  line L14 (-136.0856, 59.9795) -> (-132.2151, 59.757) construction
  line L15 (-132.2151, 59.757) -> (-130.3466, 60.4688) construction
  spline S0 degree 4 poles (-130.3466, 60.4688) (-131.8592, 61.67) (-134.662, 63.4496) (-137.4648, 64.7842) (-139.2888, 65.4071) (-141.5577, 65.6295) (-144.2716, 65.2736) (-144.6275, 64.4728) (-142.581, 62.7378) (-139.3333, 61.0472) (-136.0856, 59.9795) (-132.2151, 59.757) (-130.3466, 60.4688) knots 1 1 1 1 1 2 3 4 5 6 7 8 9 10 10 10 10 10
  point P0 (-100.2607, 79.2979)
  point P1 (0, 0)
  constraints: 4 other
extrude "Extrusion4" cut sketch "Sketch4" against normal blind 2.54
sketch "Sketch5" plane through (0, 2.54, 0) normal (0, 1, 0) x (1, 0, 0)
  spline S0 degree 4 poles (-171.6798, 20.7458) (-170.7667, 22.157) (-170.3522, 22.9696) (-169.7328, 23.9269) (-169.4633, 24.867) (-168.5064, 25.3101) (-166.5641, 25.3101) (-164.994, 25.4855) (-163.9423, 25.4855) (-161.9667, 26.3152) (-160.5355, 26.7374) (-159.7617, 27.3215) (-158.9723, 27.3215) (-158.3016, 26.4328) (-157.9485, 25.2358) (-158.507, 24.6712) (-159.147, 24.0243) knots 0 0 0 0 0 0.076923 0.153846 0.230769 0.307692 0.384615 0.461538 0.538462 0.615385 0.692308 0.769231 0.846154 0.923077 1 1 1 1 1 projected
  spline S1 degree 4 poles (-159.147, 24.0243) (-160.0581, 24.0243) (-162.6103, 23.2715) (-165.3841, 22.9617) (-167.6803, 21.8983) (-169.4313, 21.3818) (-170.5284, 19.2307) (-171.1441, 17.0833) (-170.815, 14.1366) (-169.1501, 12.4896) (-166.1802, 10.5679) knots 0 0 0 0 0 0.142857 0.285714 0.428571 0.571429 0.714286 0.857143 1 1 1 1 1 projected
  spline S2 degree 4 poles (-166.1802, 10.5679) (-161.9348, 8.4027) (-156.3592, 6.8039) (-150.8595, 4.8448) (-144.0666, 2.897) (-137.5642, 1.0325) (-133.408, -0.448) (-128.5229, -2.0136) knots 0 0 0 0 0 0.25 0.5 0.75 1 1 1 1 1 projected
  spline S3 degree 3 poles (-128.5229, -2.0136) (-122.8568, -3.6384) (-116.4732, -5.1631) (-112.6705, -6.5177) knots 0 0 0 0 1 1 1 1 projected
  spline S4 degree 4 poles (-112.6705, -6.5177) (-109.8893, -7.1819) (-108.0753, -7.8281) (-107.2685, -8.3502) (-104.7195, -10.6035) (-101.7979, -13.4938) (-97.6123, -16.6542) (-94.8687, -18.4294) (-90.3146, -20.3112) (-87.6705, -21.2531) (-84.2511, -22.0698) (-81.9397, -22.0698) (-78.0678, -22.0698) (-76.4694, -22.0698) (-75.6669, -22.589) (-73.3464, -23.4157) (-72.0061, -24.2829) knots 0 0 0 0 0 0.076923 0.153846 0.230769 0.307692 0.384615 0.461538 0.538462 0.615385 0.692308 0.769231 0.846154 0.923077 1 1 1 1 1 projected
  line L0 (-205.0817, 106.0279) -> (-14.5817, 106.0279) construction
  line L1 (-14.5817, 106.0279) -> (-14.5817, -35.5241) construction
  line L2 (-14.5817, -35.5241) -> (-205.0817, -35.5241) construction
  line L3 (-205.0817, -35.5241) -> (-205.0817, 106.0279) construction
  line L4 (-158.1955, 25.2858) -> (-155.516, 29.625) construction
  line L5 (-155.516, 29.625) -> (-153.2617, 31.9894) construction
  line L6 (-153.2617, 31.9894) -> (-145.3914, 31.6555) construction
  line L7 (-145.3914, 31.6555) -> (-139.7821, 30.1036) construction
  line L8 (-139.7821, 30.1036) -> (-134.6758, 28.8473) construction
  line L9 (-134.6758, 28.8473) -> (-130.7961, 29.4016) construction
  line L10 (-130.7961, 29.4016) -> (-127.7662, 31.2491) construction
  line L11 (-127.7662, 31.2491) -> (-125.6604, 33.6526) construction
  spline S5 degree 4 poles (-158.1955, 25.2858) (-155.516, 29.625) (-153.2617, 31.9894) (-145.3914, 31.6555) (-139.7821, 30.1036) (-134.6758, 28.8473) (-130.7961, 29.4016) (-127.7662, 31.2491) (-125.6604, 33.6526) knots 1 1 1 1 1 2 3 4 5 6 6 6 6 6
  line L12 (-125.6604, 33.6526) -> (-123.5802, 33.6526) construction
  line L13 (-123.5802, 33.6526) -> (-117.9479, 30.8813) construction
  line L14 (-117.9479, 30.8813) -> (-110.8761, 25.2859) construction
  line L15 (-110.8761, 25.2859) -> (-103.2826, 18.0459) construction
  line L16 (-103.2826, 18.0459) -> (-97.6716, 11.8303) construction
  line L17 (-97.6716, 11.8303) -> (-93.1657, 6.8239) construction
  line L18 (-93.1657, 6.8239) -> (-88.5999, 1.1534) construction
  line L19 (-88.5999, 1.1534) -> (-82.4018, -5.5047) construction
  line L20 (-82.4018, -5.5047) -> (-78.1463, -11.1995) construction
  line L21 (-78.1463, -11.1995) -> (-74.5788, -16.2064) construction
  line L22 (-74.5788, -16.2064) -> (-72.7872, -19.6894) construction
  spline S6 degree 4 poles (-125.6604, 33.6526) (-123.5802, 33.6526) (-117.9479, 30.8813) (-110.8761, 25.2859) (-103.2826, 18.0459) (-97.6716, 11.8303) (-93.1657, 6.8239) (-88.5999, 1.1534) (-82.4018, -5.5047) (-78.1463, -11.1995) (-74.5788, -16.2064) (-72.7872, -19.6894) (-73.1688, -20.0371) (-73.4414, -20.2099) (-73.5691, -20.2795) knots 1 1 1 1 1 2 3 4 5 6 7 8 9 10 11 11.834077 11.834077 11.834077 11.834077 11.834077
  line L23 (-73.5691, -20.2795) -> (-73.1601, -21.6544) construction
  line L24 (-73.1601, -21.6544) -> (-73.1601, -23.619) construction
  spline S7 degree 2 poles (-73.5691, -20.2795) (-73.1601, -21.6544) (-73.1601, -23.619) knots 1 1 1 2 2 2
  line L25 (-72.7872, -19.6894) -> (-73.1688, -20.0371) construction
  line L26 (-73.1688, -20.0371) -> (-73.4414, -20.2099) construction
  line L27 (-73.4414, -20.2099) -> (-73.5691, -20.2795) construction
  point P0 (-100.2607, 79.2979)
  point P1 (-112.1882, 86.8255)
  point P2 (-139.7824, 80.7529)
  point P3 (0, 0)
  constraints: 2 parallel, 1 perpendicular, 18 other
extrude "Extrusion5" add sketch "Sketch5" along normal blind 2.54